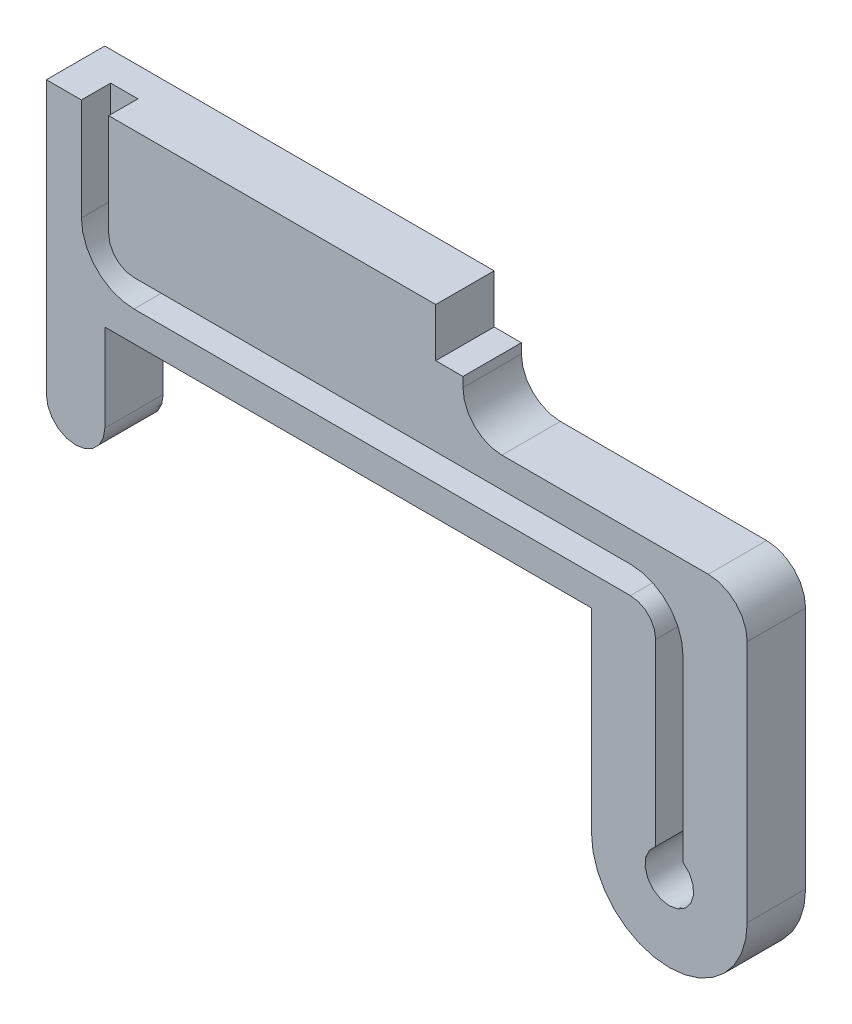
# Autodesk Inventor part: RackeSecondaryStacring
Saved by Autodesk Inventor 2019 (Build 230136000, 136)
## iProperties
Created: 2022-06-19
Part Number: RackeSecondaryStacring
Material: Типовые
Document SubType Name: Modeling
Designer: Dazer
Density: 1 g/cm^3
Appearance: По умолчанию
Author: Dazer
Autodesk Inventor part; units mm, degrees
ref_plane "YZ Plane" through (0, 0, 0) normal (1, 0, 0) x (0, 1, 0)
ref_plane "XZ Plane" through (0, 0, 0) normal (0, 1, 0) x (-1, 0, 0)
ref_plane "XY Plane" through (0, 0, 0) normal (0, 0, 1) x (1, 0, 0)
sketch "Эскиз1" plane through (0, 0, 0) normal (0, 0, 1) x (1, 0, 0)
  line L0 (-0.2, 0) -> (-0.2, 2.5)
  line L1 (-0.2, 2.5) -> (-20.2, 2.5)
  line L2 (-20.2, 0) -> (-20.2, 2.5)
  line L3 (-0.2, 0) -> (1.2, 0)
  line L4 (1.2, 0) -> (1.2, -3.5)
  line L5 (-20.2, -13) -> (-17.2, -13)
  line L6 (-17.2, -7) -> (7.8, -7)
  line L7 (7.8, -13) -> (15.8, -13)
  line L8 (15.8, -3.5) -> (1.2, -3.5)
  line L9 (7.8, -13) -> (7.8, -17)
  line L10 (15.8, -17) -> (15.8, -13)
  arc A0 (7.8, -17) -> (15.8, -17) centre (11.8, -17) ccw
  circle A1 centre (11.8, -17) radius 1.25
  line L11 (15.8, -13) -> (15.8, -3.5)
  line L12 (7.8, -7) -> (7.8, -13)
  line L13 (-17.2, -7) -> (-17.2, -13)
  line L14 (-20.2, -13) -> (-20.2, 0)
  line L15 (-6.1183, 2.5) -> (-8.8117, 2.5)
  point P0 (0, 0)
  dimension "d0" = 2.5
  constraints: 32 end point, 4 vertical, 2 centre point, 2 horizontal, 2 parallel, 2 point on circle, 1 coincident
  measures "d0" diameter of A1
extrude "Выдавливание1" add sketch "Эскиз1" along normal blind 3
sketch "Эскиз2" plane through (1.2, -3.5, 0) normal (0, 1, 0) x (1, 0, 0)
  line L0 (11.85, 0) -> (11.85, -3) projected
  line L1 (14.6, 0) -> (0, 0) projected
  line L2 (0, 0) -> (0, -3) projected
  line L3 (14.6, -3) -> (0, -3) projected
  line L4 (14.6, 0) -> (14.6, -3) projected
  point P0 (-1.2, 0)
extrude "Выдавливание2" add sketch "Эскиз2" along normal blind 1
fillet "Сопряжение1" radius 2 2 edges at (15.8, -2.5, 1.5) (1.2, -2.5, 1.5)
fillet "Сопряжение1" radius 1.5 2 edges at (-17.2, -13, 1.5) (-20.2, -13, 1.5)
sketch "Эскиз3" plane through (0, 0, 3) normal (0, 0, 1) x (1, 0, 0)
  line L0 (-18.4, 2.5) -> (-18.4, -2.75)
  arc A0 (-18.4, -2.75) -> (-15.7, -5.45) centre (-15.7, -2.75) ccw
  line L1 (-15.7, -5.45) -> (9.8, -5.45)
  arc A1 (11.1, -6.75) -> (9.8, -5.45) centre (9.8, -6.75) ccw
  line L2 (11.1, -6.75) -> (11.1, -15.75)
  line L3 (12.5, -15.75) -> (12.5, -6.75)
  arc A2 (12.5, -6.75) -> (9.8, -4.05) centre (9.8, -6.75) ccw
  line L4 (9.8, -4.05) -> (-15.7, -4.05)
  arc A3 (-17, -2.75) -> (-15.7, -4.05) centre (-15.7, -2.75) ccw
  line L5 (-17, -2.75) -> (-17, 2.5)
  line L6 (-17, 2.5) -> (-18.4, 2.5)
  line L7 (12.5, -15.75) -> (12.5, -17.0201)
  line L8 (12.5, -17.0201) -> (11.1, -17.0201)
  line L9 (11.1, -17.0201) -> (11.1, -15.75)
  point P0 (0, 0)
  constraints: 20 end point, 8 point on circle, 4 centre point, 3 perpendicular, 1 collinear, 1 vertical
extrude "Выдавливание3" cut sketch "Эскиз3" against normal blind 1.5
